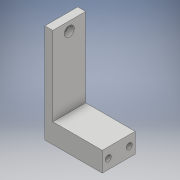
# Autodesk Inventor part: armpart4
Saved by Autodesk Inventor 2018.3 (Build 223284000, 284)
## iProperties
Created: 2019-11-01
Part Number: armpart4
Material: 一般
Document SubType Name: Modeling
Designer: Eiji Nishizawa
Density: 1 g/cm^3
Appearance: 既定
Mass: 6.57403 g
Surface Area: 32.9921 cm^2
Volume: 6.57403 cm^3
Author: Eiji Nishizawa
Autodesk Inventor part; units mm, degrees
ref_plane "YZ Plane" through (0, 0, 0) normal (1, 0, 0) x (0, 1, 0)
ref_plane "XZ Plane" through (0, 0, 0) normal (0, 1, 0) x (-1, 0, 0)
ref_plane "XY Plane" through (0, 0, 0) normal (0, 0, 1) x (1, 0, 0)
sketch "スケッチ1" plane through (0, 0, 0) normal (1, 0, 0) x (0, 1, 0)
  line L0 (7.8325, 11.4458) -> (-8.7675, 11.4458)
  line L1 (-8.7675, 11.4458) -> (-8.7675, -38.5542)
  line L2 (-8.7675, -38.5542) -> (7.8325, -38.5542)
  line L3 (7.8325, -38.5542) -> (7.8325, 11.4458)
  circle A0 centre (-0.4675, 6.9458) radius 2.5
  line L4 (7.8325, 11.4458) -> (-8.7675, 11.4458)
  line L5 (-8.7675, 11.4458) -> (-8.7675, -38.5542)
  line L6 (-8.7675, -38.5542) -> (7.8325, -38.5542)
  line L7 (7.8325, -38.5542) -> (7.8325, 11.4458)
  circle A1 centre (-0.4675, 6.9458) radius 2.5
  point P0 (0, 0)
  point P1 (0, 0)
  point P2 (0, 0)
  dimension "d0" = 16.6
  dimension "d1" = 5
  dimension "d2" = 8.3
  dimension "d3" = 8.3
  dimension "d4" = 4.5
  dimension "d5" = 2
  dimension "d6" = 50
  dimension "d7" = 16.6
  dimension "d8" = 5
  dimension "d9" = 8.3
  dimension "d10" = 8.3
  dimension "d11" = 4.5
  dimension "d12" = 2
  dimension "d13" = 50
  constraints: 16 end point, 4 parallel, 2 centre point, 2 horizontal, 2 perpendicular
  measures "d0" distance of L0.start L0.end
  measures "d1" diameter of A0
  measures "d2" distance from line of L3 A0.centre
  measures "d3" distance from line of L1 A0.centre
  measures "d4" distance from line of L0 A0.centre
  measures "d5" distance edge to line of A0 L0
  measures "d6" distance of L2.end L0.start
  measures "d7" distance of L4.start L4.end
  measures "d8" diameter of A1
  measures "d9" distance from line of L7 A1.centre
  measures "d10" distance from line of L5 A1.centre
  measures "d11" distance from line of L4 A1.centre
  measures "d12" distance edge to line of A1 L4
  measures "d13" distance of L6.end L4.start
extrude "押し出し1" add sketch "スケッチ1" along normal blind 3
sketch "スケッチ2" plane through (3, 0, 0) normal (1, 0, 0) x (0, 0, -1)
  line L0 (-11.4458, -8.7675) -> (38.5542, -8.7675) projected
  line L1 (38.5542, 7.8325) -> (-11.4458, 7.8325) projected
  line L2 (38.5542, -8.7675) -> (28.5542, -8.7675)
  line L3 (28.5542, -8.7675) -> (28.5542, 7.8325)
  line L4 (28.5542, 7.8325) -> (38.5542, 7.8325)
  line L5 (38.5542, 7.8325) -> (38.5542, -8.7675)
  point P0 (0, 0)
  dimension "d16" = 10
  constraints: 8 end point, 2 parallel, 1 horizontal, 1 perpendicular, 1 point on line
  measures "d16" distance between parallel lines of L5 L3
extrude "押し出し2" add sketch "スケッチ2" along normal blind 25
sketch "スケッチ3" plane through (0, 0, 0) normal (-1, 0, 0) x (0, 0, 1)
  line L0 (-28.5542, 7.8325) -> (11.4458, 7.8325) projected
  line L1 (-38.5542, -8.7675) -> (-38.5542, 7.8325) projected
  line L2 (11.4458, 7.8325) -> (-38.5542, 7.8325)
  line L3 (-38.5542, 7.8325) -> (-38.5542, -8.7675)
  line L4 (-38.5542, -8.7675) -> (11.4458, -8.7675)
  line L5 (11.4458, -8.7675) -> (11.4458, 7.8325)
  circle A0 centre (6.9458, -0.4675) radius 2.5 projected
  circle A1 centre (6.9458, -0.4675) radius 1.5
  point P0 (0, 0)
  dimension "d19" = 3
  constraints: 8 end point, 2 parallel, 1 centre point, 1 coincident, 1 horizontal, 1 perpendicular
  measures "d19" diameter of A1
extrude "押し出し3" add sketch "スケッチ3" along normal blind 1 contours L0 L5 L4 L1 L2 | A0
sketch "スケッチ4" plane through (28, 0, 0) normal (1, 0, 0) x (0, 0, -1)
  circle A0 centre (33.5542, -5.7675) radius 1.5
  circle A1 centre (33.5542, 4.8325) radius 1.5
  line L0 (28.5542, -8.7675) -> (38.5542, -8.7675) projected
  line L1 (38.5542, 7.8325) -> (28.5542, 7.8325) projected
  line L2 (28.5542, 7.8325) -> (28.5542, -8.7675) projected
  point P0 (0, 0)
  dimension "d22" = 3
  dimension "d23" = 3
  dimension "d24" = 3
  dimension "d25" = 3
  dimension "d26" = 5
  dimension "d27" = 5
  constraints: 2 centre point
  measures "d22" distance from line of L0 A0.centre
  measures "d23" diameter of A0
  measures "d24" distance from line of L1 A1.centre
  measures "d25" diameter of A1
  measures "d26" distance from line of L2 A0.centre
  measures "d27" distance from line of L2 A1.centre
extrude "押し出し4" cut sketch "スケッチ4" against normal blind 100
